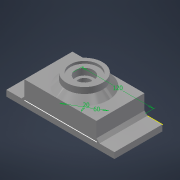
# Autodesk Inventor part: soporte de rodamientos
Saved by Autodesk Inventor 2022 (Build 260153000, 153)
## iProperties
Created: 2021-09-08
Part Number: soporte de rodamientos
Material: Stainless Steel
Document SubType Name: Modeling
Designer: Andres
Density: 8 g/cm^3
Appearance: Steel
Author: Andres
Autodesk Inventor part; units mm, degrees
ref_plane "YZ Plane" through (0, 0, 0) normal (1, 0, 0) x (0, 1, 0)
ref_plane "XZ Plane" through (0, 0, 0) normal (0, 1, 0) x (-1, 0, 0)
ref_plane "XY Plane" through (0, 0, 0) normal (0, 0, 1) x (1, 0, 0)
sketch "Sketch4" plane through (0, 0, 0) normal (0, 1, 0) x (-1, 0, 0)
  line L0 (90, 40) -> (-90, 40)
  line L1 (-90, 40) -> (-90, -40)
  line L2 (-90, -40) -> (90, -40)
  line L3 (90, -40) -> (90, 40)
  line L4 (90, 40) -> (-90, -40) construction
  line L5 (-90, 40) -> (90, -40) construction
  point P0 (0, 0)
  dimension "d26" = 180
  dimension "d27" = 80
  constraints: 12 end point, 2 midpoint, 2 parallel, 1 horizontal, 1 perpendicular
  measures "d26" distance of L2.end L1.end
  measures "d27" distance of L1.end L0.end
extrude "Extrusion5" add sketch "Sketch4" along normal blind 10
sketch "Sketch5" plane through (0, 10, 0) normal (0, 1, 0) x (1, 0, 0)
  circle A0 centre (0, 0) radius 10
  circle A1 centre (0, 0) radius 30
  line L0 (90, 40) -> (-90, 40) projected
  line L1 (60, -40) -> (-60, -40)
  line L2 (-60, -40) -> (-60, 40)
  line L3 (-60, 40) -> (60, 40)
  line L4 (60, 40) -> (60, -40)
  line L5 (60, -40) -> (-60, 40) construction
  line L6 (-60, -40) -> (60, 40) construction
  point P0 (60, 40)
  dimension "d30" = 20
  dimension "d33" = 60
  dimension "d36" = 120
  constraints: 12 end point, 2 centre point, 2 coincident, 2 midpoint, 2 parallel, 1 horizontal, 1 perpendicular, 1 point on line
  measures "d30" diameter of A0
  measures "d33" diameter of A1
  measures "d36" distance of L2.end L3.end
extrude "Extrusion6" add sketch "Sketch5" along normal blind 30 contours L4 L1 L2 L0
extrude "Extrusion7" add sketch "Sketch5" along normal blind 50 contours A1
chamfer "Chamfer2" distance 10 angle 45 1 edges at (-30, 40, 0)
chamfer "Chamfer3" distance 5 angle 45 2 edges at (60, 10, 0) (-60, 10, 0)
sketch "Sketch6" plane through (0, 60, 0) normal (0, 1, 0) x (1, 0, 0)
  circle A0 centre (0, 0) radius 15
  circle A1 centre (0, 0) radius 23.5
  circle A2 centre (0, 0) radius 10 projected
  circle A3 centre (0, 0) radius 10 projected
  dimension "d42" = 30
  dimension "d43" = 47
  constraints: 2 centre point, 2 coincident
  measures "d42" diameter of A0
  measures "d43" diameter of A1
extrude "Extrusion8" cut sketch "Sketch6" against normal blind 4 contours A1
extrude "Extrusion9" cut sketch "Sketch6" against normal blind 15 contours A0
body "Solid2"
